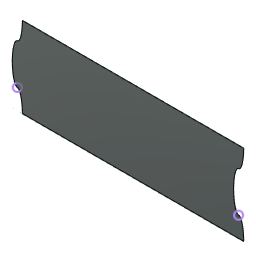
belt v2 (Autodesk Fusion 360 design; units mm, degrees)
Autodesk Fusion 360 part; units mm, degrees
sketch "Sketch1" plane through (0, 0, 0) normal (0, 0, 1) x (1, 0, 0)
  line L0 (212.5, 77.5) -> (-212.5, 77.5)
  line L1 (-212.5, 77.5) -> (-212.5, -77.5)
  line L2 (-212.5, -77.5) -> (212.5, -77.5)
  line L3 (212.5, -77.5) -> (212.5, 77.5)
  line L4 (212.5, 77.5) -> (-212.5, -77.5) construction
  line L5 (-212.5, 77.5) -> (212.5, -77.5) construction
  ellipse E0 centre (-212.5, 77.5) end of major axis (-212.5, 116.25) minor radius 9.6875
  line L6 (-212.5, 38.75) -> (-212.5, 116.25)
  line L7 (-202.8125, 77.5) -> (-222.1875, 77.5)
  ellipse E1 centre (212.5, 77.5) end of major axis (212.5, 116.25) minor radius 9.6875
  ellipse E2 centre (-212.5, 0) end of major axis (-212.5, 38.75) minor radius 9.6875
  ellipse E3 centre (212.5, 0) end of major axis (212.5, 38.75) minor radius 9.6875
  ellipse E4 centre (-212.5, -77.5) end of major axis (-212.5, -38.75) minor radius 9.6875
  ellipse E5 centre (212.5, -77.5) end of major axis (212.5, -38.75) minor radius 9.6875
  line L8 (212.5, -77.5) -> (250, -77.5)
  line L9 (212.5, 77.5) -> (250, 77.5)
  dimension "d3" = 425
  dimension "d4" = 155
  dimension "d5" = 77.5
  dimension "d6" = 19.375
  dimension "d9" = 425
  constraint horizontal L0
  constraint perpendicular L0 L1
  constraint parallel L0 L2
  constraint parallel L1 L3
  constraint coincident L4 origin
  constraint coincident L5 origin
  constraint coincident L0.end L1.start
  constraint perpendicular L0 L6
  constraint coincident E0 L6.start
  constraint coincident E0 L6.end
  constraint coincident E0 L7.start
  constraint coincident E0 L7.end
  constraint coincident L2.end L3.start
  constraint parallel L2 L8
  constraint coincident L0.start L3.end
  constraint parallel L0 L9
  measures "d3" distance of L1.end L2.end
  measures "d4" distance of L0.end L1.end
  measures "d5" distance of E0
extrude "Extrude1" add sketch "Sketch1" along normal blind 0.2 contours L0 L2 E0 E1 E2 E3 E4 E5 | L0 L3 E1 | L1 E2 | L1 E2 | L3 E1 L9 | L3 E5 L8 | L2 L3 E5
sketch "Sketch2" plane through (0, 0, 0.2) normal (0, 0, 1) x (1, 0, 0)
  line L0 (222.1875, 77.5) -> (-202.8125, 77.5)
  ellipse E0 centre (-212.5, 77.5) end of major axis (-212.5, 116.25) minor radius 9.6875 (-212.5, 38.75) -> (-202.8125, 77.5) ccw
  ellipse E1 centre (-212.5, 0) end of major axis (-212.5, 38.75) minor radius 9.6875 (-212.5, 38.75) -> (-212.5, -38.75) ccw
  ellipse E2 centre (-212.5, -77.5) end of major axis (-212.5, -38.75) minor radius 9.6875 (-202.8125, -77.5) -> (-212.5, -38.75) ccw
  line L1 (-202.8125, -77.5) -> (222.1875, -77.5)
  ellipse E3 centre (212.5, -77.5) end of major axis (212.5, -38.75) minor radius 9.6875 (222.1875, -77.5) -> (212.5, -38.75) ccw
  ellipse E4 centre (212.5, 0) end of major axis (212.5, 38.75) minor radius 9.6875 (212.5, 38.75) -> (212.5, -38.75) ccw
  ellipse E5 centre (212.5, 77.5) end of major axis (212.5, 116.25) minor radius 9.6875 (212.5, 38.75) -> (222.1875, 77.5) ccw
equation "belt_length = 425 mm"
equation "belt_width = 155 mm"
equation "d3 = belt_length"
equation "d4 = belt_width"
equation "d5 = belt_width / 2"
equation "d6 = belt_width / 8"
equation "d9 = belt_length"
equation "d10 = -belt_width"
